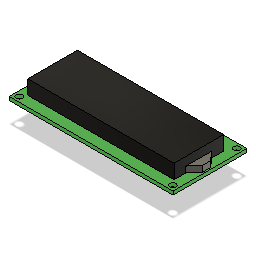
fusion-energy-monitor-case (Autodesk Fusion 360 archive; units mm, degrees)
design "Display"
Autodesk Fusion 360 part; units mm, degrees
sketch "Main PCB" plane through (0, 0, 0) normal (0, 1, 0) x (1, 0, 0)
  line L0 (12, -10) -> (92.1, -10)
  line L1 (92.1, -10) -> (92.1, -46.06)
  line L2 (92.1, -46.06) -> (12, -46.06)
  line L3 (12, -46.06) -> (12, -10)
  dimension "d1" = 80.1
  dimension "d2" = 36.06
extrude "Extrude1" add sketch "Main PCB" along normal blind 1.72 makes body 1
sketch "Display unit" plane through (0, 1.72, 0) normal (0, 1, 0) x (-1, 0, 0)
  line L0 (-12, 46.06) -> (-92.1, 46.06)
  line L1 (-92.1, 46.06) -> (-92.1, 10)
  line L2 (-92.1, 10) -> (-12, 10)
  line L3 (-12, 10) -> (-12, 46.06)
  line L4 (-16.07, 16.79) -> (-87.57, 16.79)
  line L5 (-87.57, 16.79) -> (-87.57, 41.03)
  line L6 (-87.57, 41.03) -> (-16.07, 41.03)
  line L7 (-16.07, 41.03) -> (-16.07, 16.79)
  dimension "d5" = 71.5
  dimension "d6" = 24.24
  dimension "d7" = 5.03
  dimension "d8" = 4.07
  measures "d7" distance of L0 L6
  measures "d8" distance of L3 L7
extrude "Extrude2" add sketch "Display unit" along normal blind 7 contours L4 L5 L6 L7 bodies 1
sketch "Trapezium display unit" plane through (0, 1.72, 0) normal (0, 1, 0) x (-1, 0, 0)
  line L0 (-16.07, 41.03) -> (-16.07, 16.79)
  line L1 (-16.07, 16.79) -> (-87.57, 16.79)
  line L2 (-87.57, 16.79) -> (-87.57, 41.03)
  line L3 (-87.57, 41.03) -> (-16.07, 41.03)
  line L4 (-12, 46.06) -> (-92.1, 46.06)
  line L5 (-92.1, 46.06) -> (-92.1, 10)
  line L6 (-92.1, 10) -> (-12, 10)
  line L7 (-12, 10) -> (-12, 46.06)
  line L8 (-87.57, 22.72) -> (-91.33, 26.87)
  line L9 (-91.33, 26.87) -> (-91.33, 31.07)
  line L10 (-91.33, 31.07) -> (-87.57, 35.22)
  line L11 (-87.57, 22.72) -> (-87.57, 35.22)
  dimension "d11" = 12.5
  dimension "d12" = 4.2
  dimension "d13" = 5.6
  dimension "d16" = 5.93
  measures "d16" distance of origin
extrude "Extrude3" add sketch "Trapezium display unit" along normal blind 2.9 contours L2 L8 L9 L10 L11 bodies 1
sketch "PCB holes" plane through (0, 1.72, 0) normal (0, 1, 0) x (-1, 0, 0)
  line L0 (-12, 46.06) -> (-92.1, 46.06)
  line L1 (-92.1, 46.06) -> (-92.1, 10)
  line L2 (-92.1, 10) -> (-12, 10)
  line L3 (-12, 10) -> (-12, 46.06)
  line L4 (-87.57, 22.72) -> (-91.33, 26.87)
  line L5 (-91.33, 26.87) -> (-91.33, 31.07)
  line L6 (-91.33, 31.07) -> (-87.57, 35.22)
  line L7 (-87.57, 35.22) -> (-87.57, 41.03)
  line L8 (-87.57, 41.03) -> (-16.07, 41.03)
  line L9 (-16.07, 41.03) -> (-16.07, 16.79)
  line L10 (-16.07, 16.79) -> (-87.57, 16.79)
  line L11 (-87.57, 16.79) -> (-87.57, 22.72)
  circle A0 centre (-14.48, 12.41) radius 1.5
  circle A1 centre (-89.62, 12.41) radius 1.5
  circle A2 centre (-89.62, 43.65) radius 1.5
  circle A3 centre (-14.48, 43.65) radius 1.5
  dimension "d17" = 3
  dimension "d18" = 2.41
  dimension "d19" = 2.48
  dimension "d20" = 3
  dimension "d21" = 2.41
  dimension "d22" = 2.48
  dimension "d23" = 3
  dimension "d24" = 3
  dimension "d25" = 2.48
  dimension "d26" = 2.41
  dimension "d27" = 2.48
  dimension "d28" = 2.41
  measures "d17" diameter of A0
  measures "d18" distance of L2
  measures "d19" distance of L3
  measures "d20" diameter of A1
  measures "d21" distance of L2
  measures "d22" distance of L1
  measures "d23" diameter of A2
  measures "d24" diameter of A3
  measures "d25" distance of L1 origin
  measures "d26" distance of L0 origin
  measures "d27" distance of L3
  measures "d28" distance of L0
extrude "Extrude4" cut sketch "PCB holes" against normal up to surface (1.72 mm away) contours A0 | A1 | A2 | A3 bodies 1
sketch "PINs back" plane through (0, 0, 0) normal (0, -1, 0) x (1, 0, 0)
  circle A0 centre (14.48, 43.65) radius 1.5
  circle A1 centre (89.62, 43.65) radius 1.5
  circle A2 centre (14.48, 12.41) radius 1.5
  circle A3 centre (89.62, 12.41) radius 1.5
  line L0 (92.1, 46.06) -> (12, 46.06)
  line L1 (12, 46.06) -> (12, 10)
  line L2 (12, 10) -> (92.1, 10)
  line L3 (92.1, 10) -> (92.1, 46.06)
  line L4 (18.62, 13.53) -> (59.45, 13.53)
  line L5 (59.45, 13.53) -> (59.45, 11.1)
  line L6 (59.45, 11.1) -> (18.62, 11.1)
  line L7 (18.62, 11.1) -> (18.62, 13.53)
  dimension "d31" = 40.83
  dimension "d32" = 2.43
  dimension "d33" = 1.1
  dimension "d34" = 6.62
  measures "d33" distance of L2 L6
  measures "d34" distance of L1 L7
extrude "Extrude5" add sketch "PINs back" along normal blind 3.16 contours L4 L5 L6 L7 bodies 1
sketch "PCB driver" plane through (0, -3.16, 0) normal (0, -1, 0) x (1, 0, 0)
  line L0 (18.62, 11.1) -> (59.45, 11.1)
  line L1 (59.45, 11.1) -> (59.45, 13.53)
  line L2 (59.45, 13.53) -> (18.62, 13.53)
  line L3 (18.62, 13.53) -> (18.62, 11.1)
  line L4 (17.85, 11.1) -> (59.45, 11.1)
  line L5 (59.45, 11.1) -> (59.45, 30.24)
  line L6 (59.45, 30.24) -> (17.85, 30.24)
  line L7 (17.85, 30.24) -> (17.85, 11.1)
  dimension "d37" = 41.6
  dimension "d38" = 19.14
extrude "Extrude6" add sketch "PCB driver" along normal blind 1.7 separate body makes body 2
sketch "PCB driver components" plane through (0, -4.86, 0) normal (0, -1, 0) x (1, 0, 0)
  line L0 (17.85, 30.24) -> (17.85, 11.1)
  line L1 (17.85, 11.1) -> (59.45, 11.1)
  line L2 (59.45, 11.1) -> (59.45, 30.24)
  line L3 (59.45, 30.24) -> (17.85, 30.24)
  line L4 (25.17, 23.74) -> (32.17, 23.74)
  line L5 (32.17, 23.74) -> (32.17, 16.74)
  line L6 (32.17, 16.74) -> (25.17, 16.74)
  line L7 (25.17, 16.74) -> (25.17, 23.74)
  line L8 (17.95, 26.3) -> (20.49, 26.3)
  line L9 (20.49, 26.3) -> (20.49, 15.95)
  line L10 (20.49, 15.95) -> (17.95, 15.95)
  line L11 (17.95, 15.95) -> (17.95, 26.3)
  line L12 (56.95, 22.27) -> (59.35, 22.27)
  line L13 (59.35, 22.27) -> (59.35, 17.17)
  line L14 (59.35, 17.17) -> (56.95, 17.17)
  line L15 (56.95, 17.17) -> (56.95, 22.27)
  line L16 (36.79, 25.94) -> (44.22, 25.94)
  line L17 (44.22, 25.94) -> (44.22, 15.38)
  line L18 (44.22, 15.38) -> (36.79, 15.38)
  line L19 (36.79, 15.38) -> (36.79, 25.94)
  dimension "d42" = 7
  dimension "d43" = 7
  dimension "d45" = 6.5
  dimension "d46" = 27.28
  dimension "d49" = 2.54
  dimension "d50" = 10.35
  dimension "d51" = 3.94
  dimension "d52" = 0.1
  dimension "d55" = 5.1
  dimension "d56" = 2.4
  dimension "d57" = 7.97
  dimension "d58" = 0.1
  dimension "d61" = 7.43
  dimension "d63" = 10.56
  dimension "d64" = 4.3
  dimension "d65" = 4.62
  measures "d42" distance of origin
  measures "d43" distance of L5 L7
  measures "d45" distance of L3 L4
  measures "d46" distance of L2 L5
  measures "d49" distance of origin
  measures "d50" distance of L8 L10
  measures "d51" distance of L3 L8
  measures "d52" distance of L0 L11
  measures "d55" distance of origin
  measures "d57" distance of L3 L12
  measures "d58" distance of L2 L13
  measures "d61" distance of L17 L19
  measures "d63" distance of L16 L18
  measures "d64" distance of L3 L16
  measures "d65" distance of L5 L19
extrude "Extrude10" add sketch "PCB driver components" along normal blind 2.52 contours L16 L17 L18 L19 bodies 2
extrude "Extrude9" add sketch "PCB driver components" along normal blind 3 contours L12 L13 L14 L15 bodies 2
extrude "Extrude8" add sketch "PCB driver components" along normal blind 2.9 contours L8 L9 L10 L11 bodies 2
extrude "Extrude7" add sketch "PCB driver components" along normal blind 5.1 contours L4 L5 L6 L7 bodies 2
equation "d18 = 0.91 mm + d17 / 2"
equation "d19 = 0.98 mm + d17 / 2"
equation "d20 = d17"
equation "d21 = d18"
equation "d22 = d19"
equation "d23 = d17"
equation "d24 = d17"
equation "d25 = d19"
equation "d26 = d18"
equation "d27 = d19"
equation "d28 = d18"

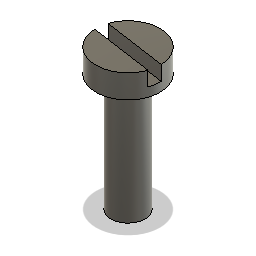
design "SCREW-MACK-M3-10MM-C2"
Autodesk Fusion 360 part; units mm, degrees
sketch "Sketch1" plane through (0, 0, 0) normal (0, 1, 0) x (1, 0, 0)
  circle A0 centre (12.1692, -9.7697) radius 2.725
  dimension "d349" = 5.45
  measures "d349" diameter of A0
extrude "Extrude1" add sketch "Sketch1" along normal blind 2
sketch "Sketch2" plane through (0, 2, 0) normal (0, 1, 0) x (-1, 0, 0)
  circle A0 centre (-12.1692, 9.7697) radius 2.725
  circle A1 centre (-12.1692, 9.7697) radius 1.455
  dimension "d352" = 2.91
  measures "d352" diameter of A1
extrude "Extrude2" add sketch "Sketch2" along normal blind 10 contours A1
sketch "Sketch3" plane through (0, 0, 0) normal (0, -1, 0) x (1, 0, 0)
  circle A0 centre (12.1692, 9.7697) radius 2.725
  line L0 (17.331, 9.2697) -> (7.0075, 9.2697)
  line L1 (7.0075, 9.2697) -> (7.0075, 10.2697)
  line L2 (7.0075, 10.2697) -> (17.331, 10.2697)
  line L3 (17.331, 10.2697) -> (17.331, 9.2697)
  line L4 (17.331, 9.2697) -> (7.0075, 10.2697) construction
  line L5 (7.0075, 9.2697) -> (17.331, 10.2697) construction
  dimension "d355" = 1
extrude "Extrude3" cut sketch "Sketch3" against normal blind 1.25 contours A0 L0 L2
move_body "Move1" bodies 1 to x (0.989838, 0, 0.142201) y (0, -1, 0) z (0.142201, 0, -0.989838) at (-1.2656, 4, 17.7096)
move_body "Move2" bodies 1 to x (1, 0, 0) y (0, 1, 0) z (0, 0, 1) at (0, 8, 0)
sketch "Sketch5" plane through (0, 12, 0) normal (0, 1, 0) x (-1, 0, 0)
  line L0 (-14.7497, 10.6455) -> (-9.4466, 9.8837)
  arc A0 (-9.4466, 9.8837) -> (-14.7497, 10.6455) centre (-12.1692, 9.7697) ccw
  circle A1 centre (-12.1692, 9.7697) radius 2.725

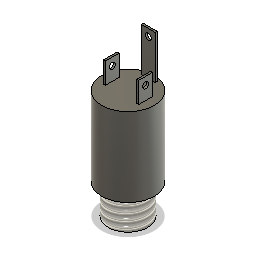
design "Gold headphone jack"
Autodesk Fusion 360 part; units mm, degrees
sketch "Jack base" plane through (0, 0, 0) normal (0, 1, 0) x (1, 0, 0)
  circle A0 centre (25, -20) radius 1.77
  circle A1 centre (25, -20) radius 2.885
  dimension "d1" = 5.77
  dimension "d2" = 3.54
  measures "d1" diameter of A1
  measures "d2" diameter of A0
extrude "Extrude1" add sketch "Jack base" along normal blind 4.45
sketch "Housing" plane through (0, 4.45, 0) normal (0, 1, 0) x (-1, 0, 0)
  circle A0 centre (-25, 20) radius 1.77
  circle A1 centre (-25, 20) radius 2.885
  circle A2 centre (-25, 20) radius 3.865
  dimension "d5" = 7.73
  measures "d5" diameter of A2
extrude "Extrude2" add sketch "Housing" along normal blind 11.67 contours A0 | A1 | A2
thread "Thread1" "ISO Metric profile 6.0 M6x1 6g" major diameter 5.884 minor diameter 4.7435 pitch 1 angle 60 resizes the face on face at (27.8707, 2.9667, 20.2873)
sketch "Pins" plane through (0, 16.12, 0) normal (0, 1, 0) x (-1, 0, 0)
  circle A0 centre (-25, 20) radius 3.865
  line L0 (-18.2729, 16.135) -> (-31.9251, 16.135) construction
  line L1 (-26.025, 17.0035) -> (-23.975, 17.0035)
  line L2 (-23.975, 17.0035) -> (-23.975, 16.7135)
  line L3 (-23.975, 16.7135) -> (-26.025, 16.7135)
  line L4 (-26.025, 16.7135) -> (-26.025, 17.0035)
  line L5 (-26.025, 17.0035) -> (-23.975, 16.7135) construction
  line L6 (-23.975, 17.0035) -> (-26.025, 16.7135) construction
  line L7 (-25, 24.5533) -> (-25, 15.4467) construction
  line L8 (-18.8718, 20) -> (-31.1282, 20) construction
  line L9 (-27.62, 21.025) -> (-27.33, 21.025)
  line L10 (-27.33, 21.025) -> (-27.33, 18.975)
  line L11 (-27.33, 18.975) -> (-27.62, 18.975)
  line L12 (-27.62, 18.975) -> (-27.62, 21.025)
  line L13 (-27.62, 21.025) -> (-27.33, 18.975) construction
  line L14 (-27.33, 21.025) -> (-27.62, 18.975) construction
  line L15 (-22.67, 21.025) -> (-22.38, 21.025)
  line L16 (-22.38, 21.025) -> (-22.38, 18.975)
  line L17 (-22.38, 18.975) -> (-22.67, 18.975)
  line L18 (-22.67, 18.975) -> (-22.67, 21.025)
  line L19 (-22.67, 21.025) -> (-22.38, 18.975) construction
  line L20 (-22.38, 21.025) -> (-22.67, 18.975) construction
  dimension "d16" = 2.05
  dimension "d17" = 0.29
  dimension "d18" = 0.29
  dimension "d19" = 0.29
  dimension "d20" = 2.05
  dimension "d21" = 2.05
  dimension "d24" = 2.33
  dimension "d25" = 2.33
  measures "d20" distance of origin
  measures "d21" distance of origin
  measures "d24" distance of L7 L18
  measures "d25" distance of L7 L10
extrude "Extrude3" add sketch "Pins" along normal blind 6.46 contours L1 L2 L3 L4
extrude "Extrude4" add sketch "Pins" along normal blind 3.11 contours L9 L10 L11 L12 | L15 L16 L17 L18
sketch "Holes in small pins" plane through (22.38, 0, 0) normal (-1, 0, 0) x (0, 0, 1)
  line L0 (18.975, 16.12) -> (21.025, 16.12)
  line L1 (21.025, 16.12) -> (21.025, 19.23)
  line L2 (21.025, 19.23) -> (18.975, 19.23)
  line L3 (18.975, 19.23) -> (18.975, 16.12)
  circle A0 centre (19.9977, 18.1) radius 0.45
  line L4 (18, 18.55) -> (23, 18.55) construction
  dimension "d30" = 0.9
  dimension "d32" = 0.68
  measures "d30" diameter of A0
  measures "d32" distance of L2 L4
extrude "Extrude5" cut sketch "Holes in small pins" against normal up to surface (5.24 mm away) contours A0
sketch "Hole in big pin" plane through (0, 0, 17.0035) normal (0, 0, 1) x (1, 0, 0)
  line L0 (23.975, 16.12) -> (26.025, 16.12)
  line L1 (26.025, 16.12) -> (26.025, 22.58)
  line L2 (26.025, 22.58) -> (23.975, 22.58)
  line L3 (23.975, 22.58) -> (23.975, 16.12)
  circle A0 centre (25.0227, 21.53) radius 0.45
  line L4 (21, 21.98) -> (31, 21.98) construction
  dimension "d35" = 0.9
  dimension "d36" = 0.6
  measures "d35" diameter of A0
  measures "d36" distance of L2 L4
extrude "Extrude6" cut sketch "Hole in big pin" against normal up to surface (0.29 mm away) contours A0
equation "d18 = d17"
equation "d19 = d17"
equation "d20 = d16"
equation "d21 = d16"
